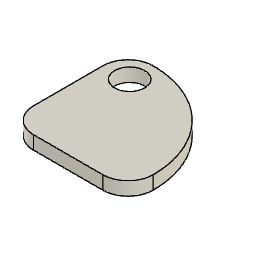
smartie_arm (Autodesk Fusion 360 design; units mm, degrees)
Autodesk Fusion 360 part; units mm, degrees
sketch "Sketch1" plane through (0, 0, 0) normal (0, 0, 1) x (1, 0, 0)
  line L0 (0, 0) -> (71.5, 0)
  line L1 (71.5, 0) -> (71.5, 71.5)
  line L2 (71.5, 71.5) -> (0, 71.5)
  line L3 (0, 71.5) -> (0, 0)
  dimension "d6" = 71.5
  dimension "d15" = 71.5
  constraint horizontal L0
  constraint vertical L1
  constraint horizontal L2
  constraint vertical L3
  constraint coincident L0.start L3.end
  measures "d6" distance of L1.end L2.end
  measures "d15" distance of L0.end L1.end
extrude "Extrude1" add sketch "Sketch1" along normal blind 8
sketch "Sketch3" plane through (0, 0, 8) normal (0, 0, 1) x (-1, 0, 0)
  line L0 (0, -71.5) -> (0, 0)
  line L1 (0, 0) -> (-71.5, 0)
  line L2 (-71.5, 0) -> (-71.5, -71.5)
  line L3 (-71.5, -71.5) -> (0, -71.5)
  circle A0 centre (-15, -57.5) radius 9
  dimension "d5" = 18
  dimension "d8" = 15
  dimension "d9" = 56.5
  dimension "d14" = 14
  measures "d5" diameter of A0
  measures "d8" distance of L0 A0.centre
  measures "d9" distance of L2 A0.centre
  measures "d14" distance of L3 A0.centre
extrude "Extrude2" cut sketch "Sketch3" against normal blind 8 contours A0
fillet "Fillet1" radius 15 2 edges at (71.5, 71.5, 4) (0, 71.5, 4)
fillet "Fillet2" radius 15 2 edges at (0, 0, 4) (71.5, 0, 4)
sketch "Sketch4" plane through (0, 0, 8) normal (0, 0, 1) x (-1, 0, 0)
  arc A0 (-56.5, 0) -> (-71.5, -15) centre (-56.5, -15) ccw
  line L0 (-71.5, -15) -> (-71.5, -56.5)
  arc A1 (-71.5, -56.5) -> (-56.5, -71.5) centre (-56.5, -56.5) ccw
  line L1 (-56.5, -71.5) -> (-15, -71.5)
  arc A2 (-15, -71.5) -> (0, -56.5) centre (-15, -56.5) ccw
  line L2 (0, -56.5) -> (0, -15)
  arc A3 (0, -15) -> (-15, 0) centre (-15, -15) ccw
  line L3 (-15, 0) -> (-56.5, 0)
  circle A4 centre (-15, -57.5) radius 9
  circle A5 centre (-15, -15) radius 56.5
  dimension "d16" = 15
  dimension "d17" = 15
  dimension "d18" = 113
  measures "d16" horizontal distance of L2.end A3.centre
  measures "d17" distance of L3 A3.centre
  measures "d18" diameter of A5
extrude "Extrude3" cut sketch "Sketch4" against normal blind 8 contours L0 A1 L1 A5
equation "d14 = 16 mm - 2 mm"
equation "d18 = ( ( 71.5 - 15 ) * 2 ) * 1 mm"
named bodies: "Smartie Arm"
